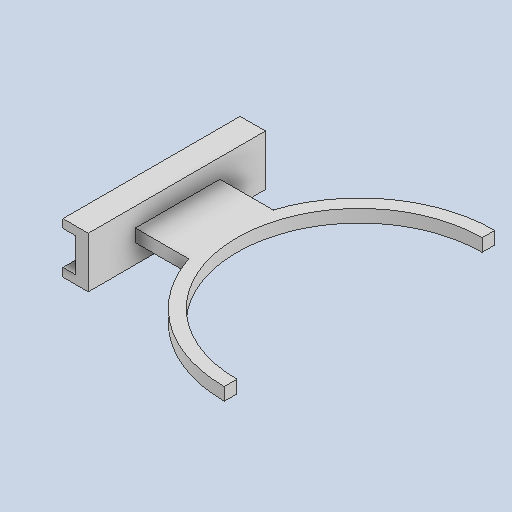
# Autodesk Inventor part: holder
Saved by Autodesk Inventor 2025 (Build 290162000, 162)
## iProperties
Created: 2025-08-07
Part Number: holder
Material: Generic
Document SubType Name: Modeling
Designer: Pravoslav
Density: 1 g/cm^3
Appearance: Default
Author: Pravoslav
Autodesk Inventor part; units mm, degrees
ref_plane "YZ Plane" through (0, 0, 0) normal (1, 0, 0) x (0, 1, 0)
ref_plane "XZ Plane" through (0, 0, 0) normal (0, 1, 0) x (-1, 0, 0)
ref_plane "XY Plane" through (0, 0, 0) normal (0, 0, 1) x (1, 0, 0)
sketch "Sketch1" plane through (0, 0, 0) normal (0, 1, 0) x (-1, 0, 0)
  circle A0 centre (0, 0) radius 14.5
  circle A1 centre (0, 0) radius 16
  line L0 (0, 16) -> (0, -16)
  line L1 (14.5, 5.0206) -> (21.5, 5.0206)
  line L2 (21.5, 5.0206) -> (21.5, -4.9794)
  line L3 (21.5, -4.9794) -> (14.5, -4.9794)
  line L4 (14.5, -4.9794) -> (14.5, 5.0206)
  point P0 (14.5, 0.0206)
  point P1 (15.2054, -4.9794)
  point P2 (15.1919, 5.0206)
  point P3 (0, 14.5)
  point P4 (0, -14.5)
  dimension "d0" = 29
  dimension "d1" = 32
  dimension "d2" = 5
  dimension "d13" = 7
  constraints: 10 end point, 2 centre point, 2 coincident, 2 parallel, 2 point on circle, 1 horizontal, 1 midpoint, 1 perpendicular, 1 vertical
  measures "d0" diameter of A0
  measures "d1" diameter of A1
  measures "d2" distance from line of L1 point (14.5, 0.021)
  measures "d13" distance between parallel lines of L2 L4
extrude "Extrusion1" add sketch "Sketch1" along normal blind 1.5 contours L4 L3 A1 L0 A0 | L4 L1 A1 L3 | A0 L0 A1 L1 L4 | A1 L1 L2 L3
sketch "Sketch2" plane through (-21.5, 0, -4.9794) normal (-1, 0, 0) x (0, 0, 1)
  line L0 (-5.3921, 3.75) -> (15.5709, 3.75)
  line L1 (15.5709, 3.75) -> (15.5709, -2.25)
  line L2 (15.5709, -2.25) -> (-5.3921, -2.25)
  line L3 (-5.3921, -2.25) -> (-5.3921, 3.75)
  line L4 (0, 0) -> (0, 1.5) projected
  point P0 (4.9794, 0)
  point P1 (5.0894, 3.75)
  point P2 (0, 0.75)
  dimension "d5" = 6
  dimension "d6" = 3
  constraints: 8 end point, 2 midpoint, 2 parallel, 1 horizontal, 1 perpendicular
  measures "d5" distance from line of L2 point (5.089, 3.75)
  measures "d6" distance from line of L0 point (0, 0.75)
extrude "Extrusion2" add sketch "Sketch2" along normal blind 1.5
sketch "Sketch3" plane through (-23, 0, -4.9794) normal (-1, 0, 0) x (0, 0, 1)
  line L0 (15.5709, 3.75) -> (-5.3921, 3.75) projected
  line L1 (15.5709, -2.25) -> (15.5709, 3.75) projected
  line L2 (-5.3921, 3.75) -> (15.5709, 3.75)
  line L3 (15.5709, 3.75) -> (15.5709, 2.75)
  line L4 (15.5709, 2.75) -> (-5.3921, 2.75)
  line L5 (-5.3921, 2.75) -> (-5.3921, 3.75)
  line L6 (-5.3921, -2.25) -> (15.5709, -2.25)
  line L7 (15.5709, -2.25) -> (15.5709, -1.25)
  line L8 (15.5709, -1.25) -> (-5.3921, -1.25)
  line L9 (-5.3921, -1.25) -> (-5.3921, -2.25)
  point P0 (4.9794, 0)
  point P1 (15.5709, -2.25)
  dimension "d9" = 1
  dimension "d10" = 1
  constraints: 16 end point, 4 parallel, 3 point on line, 2 horizontal, 2 perpendicular
  measures "d9" distance of L2.end L3.end
  measures "d10" distance of L7.end L6.end
extrude "Extrusion3" add sketch "Sketch3" along normal blind 1.5
body "Solid1"
